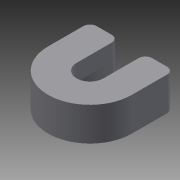
# Autodesk Inventor part: HeadConnector
Saved by Autodesk Inventor 2014 SP1 (Build 180222100, 222)
## iProperties
Created: 2013-10-30
Part Number: HeadConnector
Material: Generic
Document SubType Name: Modeling
Designer: david
Density: 1 g/cm^3
Appearance: Default
HeadConnectorDiam: 8,000 mm
HeadConnectorHeight: 2,000 mm
HeadConnectorOuterSize: 10,000 mm
HeadConnectorWidth: 3,200 mm
HeadConnectorOuterHeight: 2,000 mm
HeadConnectorTolerance: 0,200 mm
HeadConnectorProportion: 0,400 ul
Author: david
Autodesk Inventor part; units mm, degrees
ref_plane "YZ Plane" through (0, 0, 0) normal (1, 0, 0) x (0, 1, 0)
ref_plane "XZ Plane" through (0, 0, 0) normal (0, 1, 0) x (-1, 0, 0)
ref_plane "XY Plane" through (0, 0, 0) normal (0, 0, 1) x (1, 0, 0)
sketch "Sketch1" plane through (0, 0, 0) normal (0, 1, 0) x (-1, 0, 0)
  arc A0 (5, 0) -> (-5, 0) centre (0, 0) ccw
  arc A1 (1.6, 0) -> (-1.6, 0) centre (0, 0) ccw
  line L0 (-5, 0) -> (5, 0) construction
  line L1 (0, 0) -> (0, 11.6178) construction
  line L2 (-5, 0) -> (-5, -5)
  line L3 (-1.6, 0) -> (-1.6, -5)
  line L4 (1.6, 0) -> (1.6, -5)
  line L5 (5, 0) -> (5, -5)
  line L6 (-5, -5) -> (-1.6, -5)
  line L7 (1.6, -5) -> (5, -5)
  dimension "d0" = 10
  dimension "d2" = 5
  dimension "d3" = 3.2
  dimension "d6" = 5
  dimension "d8" = 5
  constraints: 16 end point, 4 point on circle, 4 tangent, 3 parallel, 2 centre point, 2 coincident, 2 point on line, 1 horizontal, 1 perpendicular
  measures "d0" distance of L0.end L0.start
  measures "d2" radius of A0
  measures "d3" distance of L3.start L4.start
  measures "d6" distance of L2.end L0.start
  measures "d8" distance from line of L1.end L5
extrude "Extrusion1" add sketch "Sketch1" against normal blind 2
sketch "Sketch2" plane through (0, -2, 0) normal (0, -1, 0) x (1, 0, 0)
  arc A0 (5, 0) -> (-5, 0) centre (0, 0) ccw projected
  line L0 (-5, 0) -> (-5, -5) projected
  line L1 (-1.6, -5) -> (-1.6, 0) projected
  arc A1 (1.6, 0) -> (-1.6, 0) centre (0, 0) ccw projected
  line L2 (1.6, 0) -> (1.6, -5) projected
  line L3 (5, -5) -> (5, 0) projected
  arc A2 (1.6, -3.6661) -> (-1.6, -3.6661) centre (0, 0) ccw
  arc A3 (5, 0) -> (-5, 0) centre (0, 0) ccw
  line L4 (-5, 0) -> (-5, -5)
  line L5 (-1.6, -5) -> (-1.6, -3.6661)
  line L6 (1.6, -3.6661) -> (1.6, -5)
  line L7 (5, -5) -> (5, 0)
  line L8 (-5, -5) -> (-1.6, -5)
  line L9 (1.6, -5) -> (5, -5)
  dimension "d11" = 4
  constraints: 12 end point, 5 point on circle, 4 tangent, 3 collinear, 2 centre point, 2 coincident, 2 point on line, 1 parallel, 1 perpendicular
  measures "d11" radius of A2
extrude "Extrusion2" add sketch "Sketch2" along normal blind 2 contours L3 L9 L2 A2 L1 L8 L0 A0
fillet "Fillet1" radius 0.8 1 edges at (5, -2, -5)
fillet "Fillet2" radius 0.8 3 edges at (1.6, -2, -5) (-1.6, -2, -5) (-5, -2, -5)
sketch "Sketch3" plane through (0, -2, 0) normal (0, -1, 0) x (1, 0, 0)
  arc A0 (1.6, -3.6661) -> (-1.6, -3.6661) centre (0, 0) ccw projected
  line L0 (-1.6, -3.6661) -> (-1.6, 0) projected
  arc A1 (1.6, 0) -> (-1.6, 0) centre (0, 0) ccw projected
  line L1 (1.6, 0) -> (1.6, -3.6661) projected
  line L2 (0, 13.9059) -> (0, -15.9339) construction
  line L3 (-15.858, 1.1715) -> (17.8906, -4.7793) construction
  line L4 (-15.3023, 4.3229) -> (18.4463, -1.6279) construction
  line L5 (-1.6, -13.7399) -> (-1.6, 21.8718) construction
  line L6 (1.6, -3.6661) -> (1.6, -1.9068)
  line L7 (3.3325, -2.2123) -> (1.6, -1.9068)
  line L8 (-3.3325, 2.2123) -> (-1.6, 1.9068)
  line L9 (-1.6, 3.6661) -> (-1.6, 1.9068)
  arc A2 (-2, 3.4641) -> (-3.3325, 2.2123) centre (0, 0) ccw
  arc A3 (1.6, -3.6661) -> (3.3325, -2.2123) centre (0, 0) ccw
  dimension "d27" = 80
  constraints: 16 end point, 7 point on circle, 7 point on line, 3 collinear, 3 parallel, 2 centre point, 2 coincident, 2 tangent
  measures "d27" angle of L2 L4
extrude "Extrusion3" add sketch "Sketch3" along normal blind 2 contours L1 L7 A0 | L9 L8 A0
equation "\"d0\" = HeadConnectorOuterSize"
equation "\"d2\" = 0.5 * HeadConnectorOuterSize"
equation "\"d3\" = HeadConnectorWidth"
equation "\"d6\" = 0.5 * HeadConnectorOuterSize"
equation "\"d8\" = 0.5 * HeadConnectorOuterSize"
equation "\"d9\" = HeadConnectorOuterHeight"
equation "\"d11\" = 0.5 * HeadConnectorDiam"
equation "\"d12\" = HeadConnectorHeight"
equation "\"d14\" = 2 * HeadConnectorProportion"
equation "\"d15\" = 2 * HeadConnectorProportion"
equation "\"d28\" = HeadConnectorHeight"
equation "\"HeadConnectorDiam\" = 20 * HeadConnectorProportion"
equation "\"HeadConnectorWidth\" = 8 * HeadConnectorProportion"
equation "\"HeadConnectorOuterSize\" = 25 * HeadConnectorProportion"
equation "\"HeadConnectorHeight\" = 5 * HeadConnectorProportion"
equation "\"HeadConnectorOuterHeight\" = 5 * HeadConnectorProportion"
equation "\"HeadConnectorTolerance\" = 0.2"
equation "\"HeadConnectorProportion\" = 0.4"
body "Solid1"
